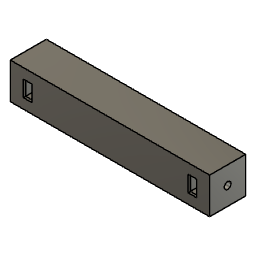
psu_brace (Autodesk Fusion 360 design; units mm, degrees)
Autodesk Fusion 360 part; units mm, degrees
sketch "brace" plane through (0, 0, 0) normal (0, 1, 0) x (1, 0, 0)
  line L0 (0, 0) -> (-83, 0)
  line L1 (-83, 0) -> (-83, 15)
  line L2 (-83, 15) -> (0, 15)
  line L3 (0, 15) -> (0, 0)
  dimension "d1" = 83
  dimension "d2" = 15
  constraint horizontal L0
  constraint vertical L1
  constraint horizontal L2
  constraint vertical L3
  constraint coincident L0.start L3.end
  measures "d1" distance of L0.start L0.end
  measures "d2" distance of L0.start L2.end
extrude "Extrude1" add sketch "brace" along normal blind 15
sketch "3mm hole" plane through (0, 0, 0) normal (1, 0, 0) x (0, 0, -1)
  line L0 (15, 0) -> (0, 0) construction
  line L1 (7.5, 0) -> (7.5, 7.5) construction
  circle A0 centre (7.5, 7.5) radius 1.425
  dimension "d5" = 7.5
  dimension "d6" = 2.85
  constraint midpoint L0 L1.start
  constraint perpendicular L0 L1
  constraint coincident L1.end A0.centre
  measures "d5" distance of L1.start L1.end
  measures "d6" diameter of A0
sketch "side nut slot" plane through (0, 0, 0) normal (0, 0, 1) x (1, 0, 0)
  line L0 (0, 0) -> (-5.9, 0) construction
  line L1 (-5.9, 0) -> (-5.9, 4.65) construction
  line L2 (-5.9, 4.65) -> (-8.5, 4.65)
  line L3 (-8.5, 4.65) -> (-8.5, 10.35)
  line L4 (-8.5, 10.35) -> (-5.9, 10.35)
  line L5 (-5.9, 10.35) -> (-5.9, 4.65)
  line L6 (-83, 0) -> (-77.1, 0) construction
  line L7 (-77.1, 0) -> (-77.1, 4.65) construction
  line L8 (-77.1, 4.65) -> (-74.5, 4.65)
  line L9 (-74.5, 4.65) -> (-74.5, 10.35)
  line L10 (-74.5, 10.35) -> (-77.1, 10.35)
  line L11 (-77.1, 10.35) -> (-77.1, 4.65)
  point P0 (-83, 0)
  dimension "d7" = 5.9
  dimension "d8" = 4.65
  dimension "d9" = 2.6
  dimension "d10" = 5.7
  dimension "d11" = 5.9
  dimension "d12" = 4.65
  dimension "d13" = 2.6
  dimension "d14" = 5.7
  constraint coincident L0.start origin
  constraint horizontal L0
  constraint perpendicular L0 L1
  constraint horizontal L2
  constraint vertical L3
  constraint horizontal L4
  constraint vertical L5
  constraint coincident P0 L6.start
  constraint perpendicular L6 L7
  constraint horizontal L8
  constraint vertical L9
  constraint horizontal L10
  constraint vertical L11
  measures "d7" distance of L0.start L0.end
  measures "d8" distance of L0.end L1.end
  measures "d9" distance of L1.end L2.end
  measures "d10" distance of L1.end L4.end
  measures "d11" distance of P0 L6.end
  measures "d12" distance of L6.end L7.end
  measures "d13" distance of L7.end L8.end
  measures "d14" distance of L7.end L10.end
extrude "Extrude2" cut sketch "side nut slot" against normal blind 12
extrude "Extrude3" cut sketch "3mm hole" against normal blind 10
extrude "Extrude4" cut sketch "3mm hole" along normal blind 10 from surface at -83
chamfer "Chamfer1" distance 0.5 angle 45 4 edges at (-77.1, 7.5, 0) (-75.8, 10.35, 0) (-74.5, 7.5, 0) (-75.8, 4.65, 0)
chamfer "Chamfer2" distance 0.5 angle 45 4 edges at (-7.2, 10.35, 0) (-5.9, 7.5, 0) (-7.2, 4.65, 0) (-8.5, 7.5, 0)
named bodies: "psu_brace"
